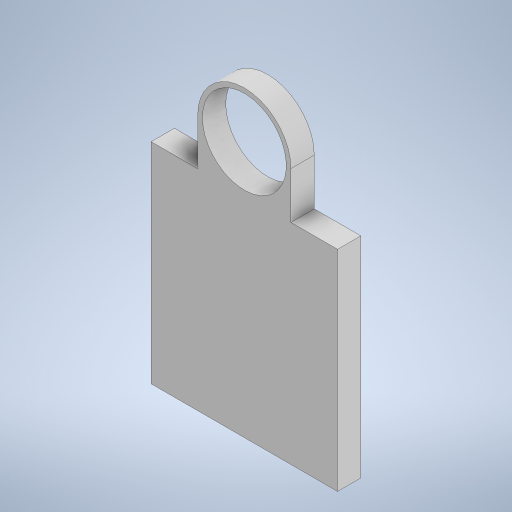
# Autodesk Inventor part: Soporte ensamble
Saved by Autodesk Inventor 2024 (Build 280153000, 153)
## iProperties
Created: 2024-03-27
Part Number: Soporte ensamble
Material: Genérico
Document SubType Name: Modeling
Designer: 50254
Density: 1 g/cm^3
Appearance: Valor por defecto
Author: 50254
Autodesk Inventor part; units mm, degrees
ref_plane "YZ Plane" through (0, 0, 0) normal (1, 0, 0) x (0, 1, 0)
ref_plane "XZ Plane" through (0, 0, 0) normal (0, 1, 0) x (-1, 0, 0)
ref_plane "XY Plane" through (0, 0, 0) normal (0, 0, 1) x (1, 0, 0)
sketch "Boceto1" plane through (0, 0, 0) normal (0, 0, 1) x (1, 0, 0)
  circle A0 centre (0, 0) radius 18
  circle A1 centre (0, 0) radius 20
  line L0 (0, -20) -> (40, -20)
  line L1 (40, -20) -> (40, -30)
  line L2 (40, -30) -> (0, -30)
  line L3 (0, -30) -> (-40, -30)
  line L4 (-40, -30) -> (-40, -20)
  line L5 (-40, -20) -> (0, -20)
  line L6 (-40, -30) -> (40, -30)
  line L7 (40, -30) -> (40, -110)
  line L8 (40, -110) -> (-40, -110)
  line L9 (-40, -110) -> (-40, -30)
  line L10 (0, 18) -> (0, -21.2387) construction
  circle A2 centre (0, 0) radius 20
  line L11 (20, 0) -> (20, -20)
  line L12 (-20, 0) -> (-20, -20)
  dimension "d0" = 36
  dimension "d1" = 40
  dimension "d2" = 40
  dimension "d3" = 10
  dimension "d4" = 40
  dimension "d5" = 80
  constraints: 26 end point, 6 perpendicular, 4 horizontal, 2 coincident, 2 midpoint, 2 parallel, 2 point on circle, 2 point on line, 1 centre point, 1 line through centre, 1 vertical alignment, 5 other
  measures "d2" distance of L0.start L0.end
  measures "d3" distance of L0.end L1.end
  measures "d4" distance of L2.end L3.end
  measures "d5" distance of L6.end L7.end
extrude "Extrusión1" add sketch "Boceto1" along normal blind 10 contours A0 | A1 | L11 L0 A1 | A1 L5 L12 | L0 L1 L2 L3 L4 L5 | L7 L8 L9 L3 L2
sketch "Boceto2" plane through (0, 0, 0) normal (0, 0, -1) x (-1, 0, 0)
  circle A0 centre (0, 0) radius 18
  dimension "d9" = 36
  constraints: 1 centre point, 1 coincident
  measures "d9" diameter of A0
hole "Agujero1" at (0, 0, 0) direction (0, 0, 1) diameter 36 depth 10 tip angle 118
